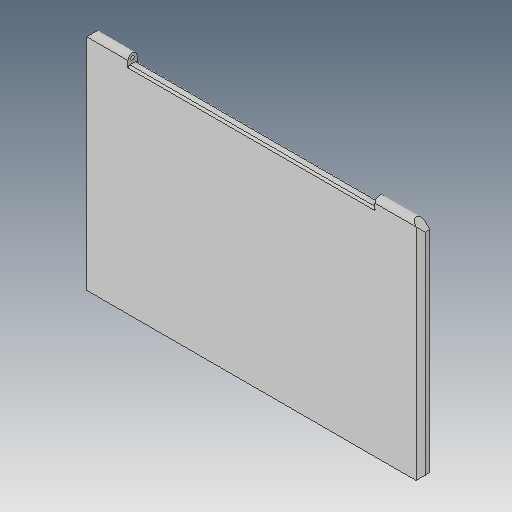
# Autodesk Inventor part: PCパーツ2
Saved by Autodesk Inventor 2020.3 (Build 243373000, 373)
## iProperties
Part Number: PCパーツ2
Material: 一般
Document SubType Name: Modeling
Designer: highs
Density: 1 g/cm^3
Appearance: 既定
Author: highs
Autodesk Inventor part; units mm, degrees
ref_plane "YZ Plane" through (0, 0, 0) normal (1, 0, 0) x (0, 1, 0)
ref_plane "XZ Plane" through (0, 0, 0) normal (0, 1, 0) x (-1, 0, 0)
ref_plane "XY Plane" through (0, 0, 0) normal (0, 0, 1) x (1, 0, 0)
sketch "スケッチ1" plane through (0, 0, 0) normal (0, 0, 1) x (1, 0, 0)
  line L0 (0, 0) -> (370, 0)
  line L1 (370, 0) -> (370, 250)
  line L2 (370, 250) -> (320, 250)
  line L3 (320, 250) -> (320, 240)
  line L4 (320, 240) -> (50, 240)
  line L5 (50, 240) -> (50, 250)
  line L6 (50, 250) -> (0, 250)
  line L7 (0, 250) -> (0, 0)
  dimension "d0" = 50
  dimension "d1" = 10
  dimension "d2" = 250
  dimension "d3" = 370
  constraints: 16 end point, 4 perpendicular, 2 point on line, 1 collinear, 1 horizontal, 1 parallel, 1 vertical
  measures "d0" distance of L5.end L6.end
  measures "d1" distance of L4.end L5.end
  measures "d2" distance of L6.end L0.start
  measures "d3" distance of L0.start L0.end
extrude "押し出し1" add sketch "スケッチ1" along normal blind 10
chamfer "面取り1" distance 5 angle 45 3 edges at (185, 0, 10) (0, 125, 10) (370, 125, 10)
chamfer "面取り2" distance 10 angle 45 4 edges at (0, 0, 2.5) (370, 0, 2.5) (370, 250, 2.5) (0, 250, 2.5)
fillet "フィレット2" radius 5 4 edges at (30, 250, 10) (30, 250, 0) (340, 250, 10) (340, 250, 0)
sketch "スケッチ2" plane through (320, 240, 0) normal (-1, 0, 0) x (0, 0, 1)
  arc A0 (10, 5) -> (0, 5) centre (5, 5) ccw projected
  circle A1 centre (5, 5) radius 2
  point P0 (0, -240)
  dimension "d14" = 4
  constraints: 1 centre point, 1 coincident
  measures "d14" diameter of A1
extrude "押し出し2" cut sketch "スケッチ2" along normal blind 280 and the other way blind 10
fillet "フィレット3" radius 2 2 edges at (185, 240, 10) (185, 240, 0)
sketch "スケッチ3" plane through (0, 0, 0) normal (0, 0, -1) x (-1, 0, 0)
  line L0 (-10, 0) -> (-360, 0) projected
  line L1 (-185, 0) -> (-185, 240) construction
  line L2 (-50, 240) -> (-320, 240) projected
  line L3 (-20, 20) -> (-350, 20)
  line L4 (-350, 20) -> (-350, 220)
  line L5 (-350, 220) -> (-20, 220)
  line L6 (-20, 220) -> (-20, 20)
  line L7 (-20, 20) -> (-350, 220) construction
  line L8 (-350, 20) -> (-20, 220) construction
  line L9 (-370, 10) -> (-370, 240) projected
  point P0 (0, 0)
  point P1 (-185, 120)
  dimension "d20" = 20
  dimension "d21" = 20
  dimension "d22" = 200
  constraints: 14 end point, 5 midpoint, 2 parallel, 2 perpendicular, 1 horizontal
  measures "d20" distance between parallel lines of L0 L3
  measures "d21" distance between parallel lines of L9 L4
  measures "d22" distance of L5.end L3.start
extrude "押し出し3" cut sketch "スケッチ3" against normal blind 1
